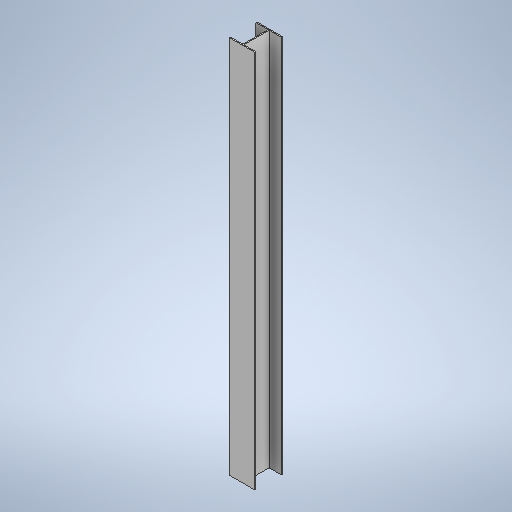
# Autodesk Inventor part: Stahlträger
Saved by Autodesk Inventor 2025.2 (Build 292293000, 293)
## iProperties
Created: 2025-02-03
Part Number: Stahlträger
Material: Generisch
Document SubType Name: Modeling
Designer: unter
Density: 1 g/cm^3
Appearance: Vorgabe
Author: unter
Autodesk Inventor part; units mm, degrees
ref_plane "YZ Plane" through (0, 0, 0) normal (1, 0, 0) x (0, 1, 0)
ref_plane "XZ Plane" through (0, 0, 0) normal (0, 1, 0) x (-1, 0, 0)
ref_plane "XY Plane" through (0, 0, 0) normal (0, 0, 1) x (1, 0, 0)
derived "Skelett_Laufkatze.ipt"
sketch "I_Traeger_front" plane through (0, 0, 0) normal (0, 1, 0) x (-1, 0, 0)
  line L0 (0, 0) -> (0, 216.8) construction
  line L1 (100, 0) -> (-100, 0)
  line L2 (-100, 0) -> (-100, 8.4)
  line L3 (-100, 8.4) -> (-4.2, 8.4)
  line L4 (-4.2, 8.4) -> (-4.2, 208.4)
  line L5 (-4.2, 208.4) -> (-100, 208.4)
  line L6 (-100, 208.4) -> (-100, 216.8)
  line L7 (-100, 216.8) -> (100, 216.8)
  line L8 (100, 216.8) -> (100, 208.4)
  line L9 (100, 208.4) -> (4.2, 208.4)
  line L10 (4.2, 208.4) -> (4.2, 8.4)
  line L11 (4.2, 8.4) -> (100, 8.4)
  line L12 (100, 8.4) -> (100, 0)
  line L13 (4.2, 208.4) -> (-4.2, 208.4) construction
sketch "I_Traeger_seite" plane through (0, 0, 0) normal (1, 0, 0) x (0, 1, 0)
  line L0 (1500, 0) -> (-1500, 0)
  line L1 (0, 8.4) -> (0, 0) construction
  line L2 (0, 208.4) -> (0, 8.4) construction
  line L3 (0, 216.8) -> (0, 208.4) construction
  line L4 (1500, 0) -> (1500, 8.4)
  line L5 (1500, 8.4) -> (-1500, 8.4)
  line L6 (-1500, 8.4) -> (-1500, 0)
  line L7 (1500, 216.8) -> (-1500, 216.8)
  line L8 (1500, 208.4) -> (-1500, 208.4)
  line L9 (-1500, 8.4) -> (-1500, 208.4)
  line L10 (-1500, 208.4) -> (-1500, 216.8)
  line L11 (1500, 8.4) -> (1500, 208.4)
  line L12 (1500, 216.8) -> (1500, 208.4)
  point P0 (0, 0)
  point P1 (0, 0)
ref_plane "Arbeitsebene1" through (0, -1500, 0) normal (0, -1, 0) x (1, 0, 0)
extrude "Extrusion1" add sketch "I_Traeger_front" along normal up to surface (3000 mm away) from surface at -1500
